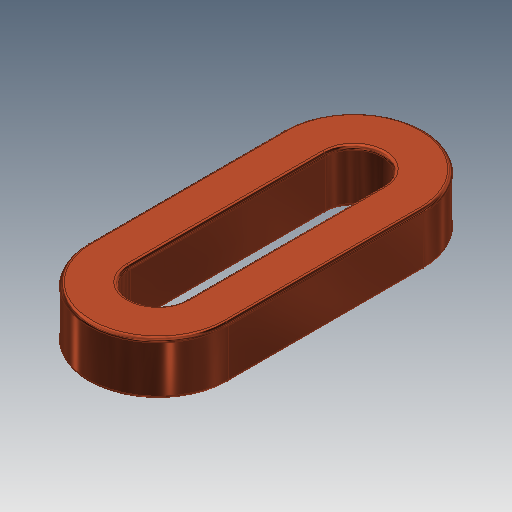
# Autodesk Inventor part: Nema 17 Coil
Saved by Autodesk Inventor 2020.2 (Build 242310000, 310)
## iProperties
Created: 2020-01-21
Part Number: Nema 17 Coil
Material: Copper
Document SubType Name: Modeling
Designer: james
Density: 8.94 g/cm^3
Appearance: Copper - Satin
Mass: 5.07092 g
Surface Area: 6.58423 cm^2
Volume: 0.567217 cm^3
Author: james
Autodesk Inventor part; units mm, degrees
ref_plane "YZ Plane" through (0, 0, 0) normal (1, 0, 0) x (0, 1, 0)
ref_plane "XZ Plane" through (0, 0, 0) normal (0, 1, 0) x (-1, 0, 0)
ref_plane "XY Plane" through (0, 0, 0) normal (0, 0, 1) x (1, 0, 0)
sketch "Sketch11" plane through (0, 0, 0) normal (0, 1, 0) x (-1, 0, 0)
  line L0 (0, 7) -> (0, -7) construction
  line L1 (-2, 7) -> (-2, -7)
  line L2 (2, -7) -> (2, 7)
  arc A0 (2, 7) -> (-2, 7) centre (0, 7) ccw
  arc A1 (-2, -7) -> (2, -7) centre (0, -7) ccw
  line L3 (5, -7) -> (5, 7)
  arc A2 (5, 7) -> (-5, 7) centre (0, 7) ccw
  line L4 (-5, 7) -> (-5, -7)
  arc A3 (-5, -7) -> (5, -7) centre (0, -7) ccw
  point P0 (0, 0)
  dimension "d82" = 14
  dimension "d83" = 10
  dimension "d84" = 3
  constraints: 12 end point, 8 point on circle, 4 centre point, 4 tangent, 2 parallel, 1 midpoint, 1 vertical, 3 other
  measures "d82" distance of L2.start L2.end
  measures "d83" distance between parallel lines of L4 L3
  measures "d84" distance between parallel lines of L2 L3
extrude "Extrusion7" add sketch "Sketch11" along normal mid plane 3.8
fillet "Fillet8" radius 0.25 16 edges at (-5, -1.9, 0) (0, -1.9, -12) (5, -1.9, 0) (0, -1.9, 12) (2, -1.9, 0) (0, -1.9, -9) (-2, -1.9, 0) (0, -1.9, 9) (5, 1.9, 0) (0, 1.9, -12) (-5, 1.9, 0) (0, 1.9, 12) (0, 1.9, -9) (2, 1.9, 0) (0, 1.9, 9) (-2, 1.9, 0)
body "Solid6"
